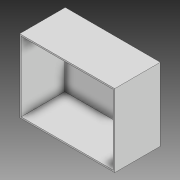
# Autodesk Inventor part: MainEnclosure
Saved by Autodesk Inventor 2020 (Build 240168000, 168)
## iProperties
Created: 2021-01-12
Part Number: MainEnclosure
Material: Generic
Document SubType Name: Modeling
Designer: DDeGo
Density: 1 g/cm^3
Appearance: Default
Author: DDeGo
Autodesk Inventor part; units mm, degrees
ref_plane "YZ Plane" through (0, 0, 0) normal (1, 0, 0) x (0, 1, 0)
ref_plane "XZ Plane" through (0, 0, 0) normal (0, 1, 0) x (-1, 0, 0)
ref_plane "XY Plane" through (0, 0, 0) normal (0, 0, 1) x (1, 0, 0)
sketch "Sketch1" plane through (0, 0, 0) normal (0, 0, 1) x (1, 0, 0)
  line L0 (-47.5, -36) -> (47.5, -36) construction
  line L1 (47.5, -36) -> (47.5, 36) construction
  line L2 (47.5, 36) -> (-47.5, 36) construction
  line L3 (-47.5, 36) -> (-47.5, -36) construction
  line L4 (-47.5, -36) -> (47.5, 36) construction
  line L5 (47.5, -36) -> (-47.5, 36) construction
  line L6 (49, -37.5) -> (-49, -37.5)
  line L7 (-49, -37.5) -> (-49, 37.5)
  line L8 (-49, 37.5) -> (49, 37.5)
  line L9 (49, 37.5) -> (49, -37.5)
  line L10 (49, -37.5) -> (-49, 37.5) construction
  line L11 (-49, -37.5) -> (49, 37.5) construction
  point P0 (0, 0)
  dimension "d0" = 72
  dimension "d1" = 95
  dimension "d2" = 1.5
  dimension "d3" = 1.5
  constraints: 24 end point, 4 midpoint, 4 parallel, 2 horizontal, 2 perpendicular
  measures "d0" distance of L2.end L0.start
  measures "d1" distance of L1.end L2.end
  measures "d2" distance between parallel lines of L8 L2
  measures "d3" distance between parallel lines of L7 L3
extrude "Extrusion1" add sketch "Sketch1" along normal blind 2
sketch "Sketch2" plane through (0, 0, 2) normal (0, 0, 1) x (1, 0, 0)
  line L0 (47.5, -36) -> (-47.5, -36)
  line L1 (-47.5, -36) -> (-47.5, 36)
  line L2 (-47.5, 36) -> (47.5, 36)
  line L3 (47.5, 36) -> (47.5, -36)
  line L4 (47.5, -36) -> (-47.5, 36) construction
  line L5 (-47.5, -36) -> (47.5, 36) construction
  line L6 (49, 37.5) -> (-49, 37.5) projected
  line L7 (-49, 37.5) -> (-49, -37.5) projected
  line L8 (-49, -37.5) -> (49, -37.5) projected
  line L9 (49, -37.5) -> (49, 37.5) projected
  point P0 (0, 0)
  constraints: 12 end point, 2 midpoint, 2 parallel, 1 coincident, 1 horizontal, 1 perpendicular
extrude "Extrusion2" add sketch "Sketch2" along normal blind 45
sketch "Sketch3" plane through (0, 0, 0) normal (0, 1, 0) x (-1, 0, 0)
  point P0 (0, 0)
body "Solid1"
